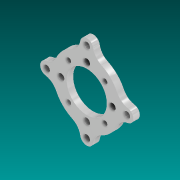
# Autodesk Inventor part: afstandsplaatje
Saved by Autodesk Inventor 2020.2 (Build 242310000, 310)
## iProperties
Created: 2020-05-15
Part Number: afstandsplaatje
Material: Aluminum 6061
Document SubType Name: Modeling
Designer: Svend
Density: 2.7 g/cm^3
Appearance: Aluminum - Polished
Author: Svend
Autodesk Inventor part; units mm, degrees
ref_plane "YZ Plane" through (0, 0, 0) normal (1, 0, 0) x (0, 1, 0)
ref_plane "XZ Plane" through (0, 0, 0) normal (0, 1, 0) x (-1, 0, 0)
ref_plane "XY Plane" through (0, 0, 0) normal (0, 0, 1) x (1, 0, 0)
sketch "Sketch1" plane through (0, 0, 0) normal (0, 0, 1) x (1, 0, 0)
  circle A0 centre (0, 0) radius 21
  circle A1 centre (16, 0) radius 2
  circle A2 centre (0, 16) radius 2
  circle A3 centre (-16, 0) radius 2
  circle A4 centre (0, -16) radius 2
  line L0 (-14.8492, -14.8492) -> (14.8492, 14.8492)
  line L1 (0, -21) -> (0, 21)
  circle A5 centre (11.3137, 11.3137) radius 1.5
  circle A6 centre (-11.3137, 11.3137) radius 1.5
  circle A7 centre (-11.3137, -11.3137) radius 1.5
  circle A8 centre (11.3137, -11.3137) radius 1.5
  circle A9 centre (0, 0) radius 12.6
  circle A10 centre (-25, 0) radius 2
  circle A11 centre (-25, 0) radius 4
  arc A12 (-25.6523, 3.9465) -> (-18.984, 8.9782) centre (-27.12, 12.826) ccw
  arc A13 (-18.984, -8.9782) -> (-25.6523, -3.9465) centre (-27.12, -12.826) ccw
  circle A14 centre (0, -25) radius 2
  circle A15 centre (0, -25) radius 4
  arc A16 (8.9782, -18.984) -> (3.9465, -25.6523) centre (12.826, -27.12) ccw
  arc A17 (-3.9465, -25.6523) -> (-8.9782, -18.984) centre (-12.826, -27.12) ccw
  circle A18 centre (25, 0) radius 2
  circle A19 centre (25, 0) radius 4
  arc A20 (18.984, 8.9782) -> (25.6523, 3.9465) centre (27.12, 12.826) ccw
  arc A21 (25.6523, -3.9465) -> (18.984, -8.9782) centre (27.12, -12.826) ccw
  circle A22 centre (0, 25) radius 2
  circle A23 centre (0, 25) radius 4
  arc A24 (-8.9782, 18.984) -> (-3.9465, 25.6523) centre (-12.826, 27.12) ccw
  arc A25 (3.9465, 25.6523) -> (8.9782, 18.984) centre (12.826, 27.12) ccw
  point P0 (18.984, -8.9782)
  point P1 (18.984, 8.9782)
  point P2 (8.9782, -18.984)
  point P3 (-8.9782, -18.984)
  point P4 (8.9782, 18.984)
  point P5 (-8.9782, 18.984)
  dimension "d0" = 42
  dimension "d1" = 4
  dimension "d5" = 16
  dimension "d8" = 360
  dimension "d10" = 45
  dimension "d11" = 3
  dimension "d12" = 16
  dimension "d15" = 360
  dimension "d19" = 25.2
  dimension "d23" = 4
  dimension "d24" = 25
  dimension "d25" = 9
  dimension "d28" = 360
  constraints: 30 point on circle, 26 centre point, 6 coincident, 5 tangent, 4 end point, 4 midpoint, 2 horizontal alignment, 1 equal radius, 1 point on line, 1 vertical, 67 other
  measures "d0" diameter of A0
  measures "d1" diameter of A1
  measures "d5" distance of point (0, 0) A1.centre
  measures "d10" angle of L1 L0
  measures "d11" diameter of A5
  measures "d12" distance of point (0, 0) A5.centre
  measures "d19" diameter of A9
  measures "d23" diameter of A10
  measures "d24" distance of point (0, 0) A10.centre
  measures "d25" radius of A12
extrude "Extrusion1" add sketch "Sketch1" along normal blind 4 contours A0 L1 A4 A9 L0 A5 | A19 A21 A0 | A0 A20 A19 | A19 | L0 A5 A9 L1 A2 A0 | A16 A15 A0 | A0 A23 A25 | A15 A17 A0 | A0 L0 A7 A9 L1 A4 | A15 | L1 A2 A9 L0 A7 A0 | A0 A24 A23 | A23 | A0 A11 A12 | A13 A11 A0 | A11
body "Solid1"
